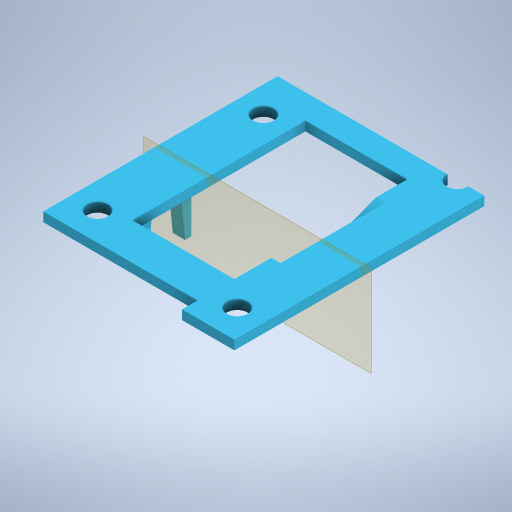
# Autodesk Inventor part: servo_und_kabelhalter
Saved by Autodesk Inventor 2023 (Build 270158000, 158)
## iProperties
Created: 2023-09-15
Part Number: servo_und_kabelhalter
Material: Generisch
Document SubType Name: Modeling
Designer: prigge
Density: 1 g/cm^3
Appearance: Türkis
Author: prigge
Autodesk Inventor part; units mm, degrees
ref_plane "YZ Plane" through (0, 0, 0) normal (1, 0, 0) x (0, 1, 0)
ref_plane "XZ Plane" through (0, 0, 0) normal (0, 1, 0) x (-1, 0, 0)
sketch "Skizze1" plane through (0, 0, 0) normal (0, 1, 0) x (-1, 0, 0)
  line L0 (0, -20) -> (33.5, -20)
  line L1 (33.5, -20) -> (33.5, 18)
  line L2 (33.5, 18) -> (0, 18)
  line L3 (0, 18) -> (0, -20)
  line L4 (-6.7, 0) -> (40.2, 0) projected
  line L5 (0, 18) -> (0, 20.5)
  line L6 (0, 20.5) -> (8.5, 20.5)
  line L7 (8.5, 20.5) -> (8.5, 18)
  line L8 (25, 12) -> (8.5, 12)
  line L9 (8.5, 12) -> (8.5, -16)
  line L10 (8.5, -16) -> (25, -16)
  line L11 (25, -16) -> (25, 12)
  point P0 (0, 0)
  dimension "d1" = 33.5
  dimension "d4" = 18
  dimension "d5" = 20
  dimension "d6" = 2.5
  dimension "d7" = 8.5
  dimension "d8" = 6
  dimension "d9" = 4
  dimension "d10" = 8.5
  dimension "d11" = 8.5
  constraints: 22 end point, 4 parallel, 4 perpendicular, 2 horizontal, 2 point on line, 1 vertical
  measures "d1" distance of L0.start L0.end
  measures "d4" distance between parallel lines of L4 L2
  measures "d5" distance between parallel lines of L0 L4
  measures "d6" distance of L6.end L7.end
  measures "d7" distance of L5.end L6.end
  measures "d8" distance between parallel lines of L2 L8
  measures "d9" distance between parallel lines of L0 L10
  measures "d10" distance between parallel lines of L3 L9
  measures "d11" distance between parallel lines of L1 L11
extrude "Extrusion1" add sketch "Skizze1" along normal blind 1.5 contours L3 L4 L9 L10 L11 L1 L0 | L3 L2 L1 L4 L11 L8 L9 | L5 L6 L7 L2
sketch "Skizze2" plane through (-8.5, 0, -16) normal (-1, 0, 0) x (0, 0, 1)
  line L0 (28, 0) -> (0, 0) projected
  line L1 (17.6, 0) -> (17.6, -5.5)
  line L2 (17.6, -5.5) -> (18.6, -5.5)
  line L3 (18.6, -5.5) -> (18.6, 0)
  line L4 (21, 0) -> (21, -5.5)
  line L5 (21, -5.5) -> (22, -5.5)
  line L6 (22, -5.5) -> (22, 0)
  line L7 (16, 2.6) -> (16, -5.1) projected
  line L8 (21, -4) -> (18.6, -4)
  line L9 (17.6, -5.5) -> (0, 0)
  point P0 (16, 0)
  point P1 (16, -5)
  dimension "d12" = 2.6
  dimension "d13" = 5
  dimension "d14" = 1
  dimension "d15" = 1
  dimension "d16" = 5.5
  dimension "d19" = 4
  constraints: 16 end point, 8 point on line, 4 perpendicular, 1 parallel, 1 vertical
  measures "d12" distance between parallel lines of L7 L3
  measures "d13" distance between parallel lines of L7 L4
  measures "d14" distance of L4.end L5.end
  measures "d15" distance of L1.end L2.end
  measures "d16" distance of L5.end L6.end
  measures "d19" distance between parallel lines of L0 L8
extrude "Extrusion2" add sketch "Skizze2" against normal blind 1.5
sketch "Skizze3" plane through (-8.5, 0, 12) normal (-1, 0, 0) x (0, 0, 1)
  line L0 (-32, 1.5) -> (6, 1.5) projected
  line L1 (-6, -5.5) -> (-6, 0) projected
  line L2 (-6, 0) -> (-28, 0) projected
  line L3 (-6, 0) -> (-6, 1.5)
  line L4 (-6, 0) -> (-6, -5.5) projected
  line L5 (-6, -3) -> (-11, -3)
  line L6 (-11, -3) -> (-23, 1.5)
  line L7 (8.5, 1.5) -> (-32, 1.5) projected
  line L8 (-9.4, -4) -> (-7, -4) projected
  line L9 (-28, 0) -> (-28, 1.5) projected
  point P0 (-12, 0)
  dimension "d20" = 1
  dimension "d21" = 5
  dimension "d23" = 5
  constraints: 6 end point, 3 point on line, 2 perpendicular
  measures "d20" distance between parallel lines of L8 L5
  measures "d21" distance from line of L9 L6.end
  measures "d23" distance of L5.start L5.end
extrude "Extrusion3" cut sketch "Skizze3" against normal up to surface (1.5 mm away) contours L0 L3 L2 L6 | L2 L1 L5 L6
sketch "Skizze4" plane through (-33.5, 0, -20) normal (-1, 0, 0) x (0, 0, 1)
  line L0 (32, 0) -> (4, 0) projected
  line L1 (16, 0) -> (16, -12)
  line L2 (16, -12) -> (17, -12)
  line L3 (17, -12) -> (17.8, -4)
  line L4 (17.8, -4) -> (20, -4)
  line L5 (20, -4) -> (20, 0)
  line L6 (20, 5.3565) -> (20, -21.6388) projected
  dimension "d26" = 3
  dimension "d27" = 2.2
  dimension "d28" = 4
  dimension "d29" = 8
  dimension "d30" = 12
  constraints: 10 end point, 2 perpendicular, 1 parallel, 1 point on line, 1 vertical
  measures "d26" distance from line of L6 L2.end
  measures "d27" distance from line of L6 L3.end
  measures "d28" distance from line of L6 L1.start
  measures "d29" distance from line of L2.end L4
  measures "d30" distance of L1.start L1.end
extrude "Extrusion4" add sketch "Skizze4" against normal blind 2
mirror "Spiegeln1" about plane through (0, 0, 0) normal (0, 0, 1) of "Extrusion4"
sketch "Skizze5" plane through (0, 1.5, 0) normal (0, 1, 0) x (1, 0, 0)
  line L0 (6.7, 0) -> (-40.2, 0) projected
  line L1 (0, -20.5) -> (0, 20) projected
  point P0 (0, 0)
  point P1 (-29.25, -13.45)
  point P2 (-29.25, 13.45)
  point P3 (-4.25, -15.8)
  point P4 (-4.25, 19.9)
  dimension "d33" = 13.45
  dimension "d34" = 13.45
  dimension "d35" = 15.8
  dimension "d36" = 19.9
  dimension "d37" = 4.25
  dimension "d38" = 29.25
  constraints: 2 vertical alignment
  measures "d33" distance from line of L0 point (-29.25, -13.45)
  measures "d34" distance from line of L0 point (-29.25, 13.45)
  measures "d35" distance from line of L0 point (-4.25, -15.8)
  measures "d36" distance from line of point (-4.25, 19.9) L0
  measures "d37" distance from line of L1 point (-4.25, 19.9)
  measures "d38" distance from line of L1 point (-29.25, 13.45)
hole "Bohrung1" at (-29.25, 1.5, 13.45) at (-29.25, 1.5, -13.45) at (-4.25, 1.5, 15.8) at (-4.25, 1.5, -19.9) direction (0, -1, 0) diameter 3.4 depth 23.75 tip angle 118
